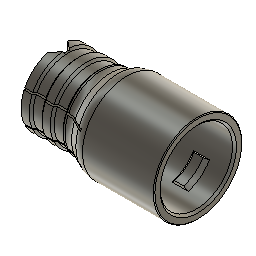
Bosch GEX 40-150 Festool Adapter v2 (Autodesk Fusion 360 design; units mm, degrees)
Autodesk Fusion 360 part; units mm, degrees
sketch "Sketch1" plane through (0, 0, 0) normal (0, 1, 0) x (1, 0, 0)
  line L0 (0, -14.25) -> (25, -14.25)
  line L1 (25, -14.25) -> (33, -18)
  line L2 (33, -18) -> (70, -18)
  line L3 (0, -14.25) -> (0, -18.25)
  line L4 (0, -18.25) -> (24.109, -18.25)
  line L5 (24.109, -18.25) -> (32.109, -22)
  line L6 (32.109, -22) -> (70, -22)
  line L7 (70, -22) -> (70, -18)
  line L8 (52, -18) -> (53.75, -16.25)
  line L9 (53.75, -16.25) -> (58.25, -16.25)
  line L10 (58.25, -16.25) -> (60, -18)
  line L11 (3.8, -5.35) -> (3.8, 5.35)
  arc A0 (3.8, 5.35) -> (0, 5.35) centre (1.9, 5.35) ccw
  line L12 (0, 5.35) -> (0, -5.35)
  arc A1 (0, -5.35) -> (3.8, -5.35) centre (1.9, -5.35) ccw
  line L13 (1.9, -7.25) -> (1.9, 7.25) construction
  line L14 (1.9, -7.25) -> (31.9, -7.25)
  line L15 (31.9, -7.25) -> (31.9, 7.25)
  line L16 (31.9, 7.25) -> (1.9, 7.25)
  line L17 (4.6, -5.35) -> (4.6, 5.35) construction
  arc A2 (4.6, 5.35) -> (-0.8, 5.35) centre (1.9, 5.35) ccw construction
  line L18 (-0.8, 5.35) -> (-0.8, -5.35) construction
  arc A3 (-0.8, -5.35) -> (4.6, -5.35) centre (1.9, -5.35) ccw construction
  line L19 (1.9, -8.05) -> (32.7, -8.05)
  line L20 (32.7, -8.05) -> (32.7, 8.05)
  line L21 (32.7, 8.05) -> (1.9, 8.05)
  line L22 (31.9, -7.25) -> (31.9, -8.05)
  line L23 (31.9, 7.25) -> (31.9, 8.05)
  line L24 (0, -14.25) -> (3.8, -10.45)
  line L25 (3.8, -10.45) -> (3.8, -14.25)
  line L26 (2.8, -11.45) -> (3.8, -11.45)
  line L27 (1.9, -8.05) -> (0, -8.05)
  line L28 (0, 8.05) -> (1.9, 8.05)
  line L29 (0, -8.05) -> (0, -5.35)
  line L30 (0, 8.05) -> (0, 5.35)
  line L31 (1.9, -7.25) -> (0, -7.25)
  line L32 (1.9, 7.25) -> (0, 7.25)
  line L33 (5, -18.25) -> (5, -17.25)
  line L34 (5, -17.25) -> (9.5, -17.25)
  line L35 (9.5, -17.25) -> (9.5, -18.25)
  line L36 (15.5, -18.25) -> (15.5, -17.25)
  line L37 (15.5, -17.25) -> (20, -17.25)
  line L38 (20, -17.25) -> (20, -18.25)
  point P0 (1.9, 0)
  dimension "d1" = 14.25
  dimension "d2" = 4
  dimension "d3" = 25
  dimension "d4" = 18
  dimension "d5" = 4
  dimension "d6" = 4
  dimension "d7" = 8
  dimension "d8" = 135
  dimension "d9" = 1.75
  dimension "d10" = 10
  dimension "d11" = 19
  dimension "d12" = 45
  dimension "d17" = 14.5
  dimension "d18" = 3.8
  dimension "d20" = 30
  dimension "d21" = 0.8
  dimension "d22" = 0.8
  dimension "d24" = 45
  dimension "d27" = 1
  dimension "d34" = 1
  dimension "d35" = 4.5
  dimension "d36" = 6
  dimension "d37" = 5
  constraint horizontal L0
  constraint parallel L0 L2
  constraint perpendicular L0 L3
  constraint perpendicular L3 L4
  constraint parallel L4 L6
  constraint vertical L7
  constraint vertical origin L0.start
  constraint parallel L1 L5
  constraint coincident L2 L8.start
  constraint parallel L2 L9
  constraint coincident L2 L10.end
  constraint equal L8 L10
  constraint tangent L11 A0
  constraint tangent A0 L12
  constraint parallel L11 L12
  constraint tangent L12 A1
  constraint tangent L11 A1
  constraint midpoint A1 L13.start
  constraint midpoint A0 L13.end
  constraint perpendicular L0 L13
  constraint midpoint L13 P0
  constraint horizontal origin P0
  constraint tangent A1 L14
  constraint perpendicular L13 L14
  constraint perpendicular L14 L15
  constraint horizontal L16
  constraint coincident L19 L22.end
  constraint perpendicular L19 L22
  constraint coincident L21 L23.end
  constraint perpendicular L21 L23
  constraint coincident origin L12
  constraint perpendicular L0 L25
  constraint coincident L0 L25.end
  constraint coincident L11 L24.end
  constraint coincident L24 L26.start
  constraint coincident L25 L26.end
  constraint perpendicular L25 L26
  constraint tangent A3 L27
  constraint parallel L19 L27
  constraint tangent A2 L28
  constraint horizontal L28
  constraint vertical L30
  constraint vertical L29
  constraint coincident L29 L31.end
  constraint coincident L30 L32.end
  constraint horizontal L32
  constraint horizontal L31
  constraint coincident L4 L33.start
  constraint perpendicular L4 L33
  constraint perpendicular L33 L34
  constraint coincident L4 L35.end
  constraint coincident L4 L36.start
  constraint perpendicular L4 L36
  constraint perpendicular L36 L37
  constraint coincident L4 L38.end
  constraint parallel L35 L38
  constraint vertical L38
  constraint equal L34 L37
  constraint equal L35 L36
  measures "d1" distance of origin L0
  measures "d2" distance of L0.start L3.end
  measures "d3" distance of L0.start L0.end
  measures "d4" distance of origin L2
  measures "d5" distance of L2 L6
  measures "d6" distance of L1 L5
  measures "d7" distance of L8.start L10.end
  measures "d8" angle of L9 L10
  measures "d9" vertical distance of L9.end L10.end
  measures "d10" distance of L2.end L10.end
  measures "d11" distance of L1.end L8.start
  measures "d12" horizontal distance of L0.end L6.end
  measures "d17" distance of L13.start L13.end
  measures "d18" distance of L11 L12
  measures "d20" distance of L13.end L15.end
  measures "d24" angle of L24 L25
  measures "d27" vertical distance of L24.end L26.start
  measures "d34" distance of L36.start L36.end
  measures "d35" distance of L36.end L37.end
  measures "d36" distance of L34.end L36.end
  measures "d37" distance of L3.end L33.start
revolve "Revolve1" add sketch "Sketch1" angle 360 about axis through (1.75, 0, 0) along (1, 0, 0) contours L0 L1 L2 L3 L4 L5 L6 L7 L33 L34 L35 L36 L37 L38 makes body 1
chamfer "Chamfer2" distance 1 angle 45 4 edges at (5, -6.5995, -17.015) (9.5, -6.5995, -17.015) (15.5, -6.5995, -17.015) (20, -6.5995, -17.015) on bodies 1
revolve "Revolve2" add sketch "Sketch1" angle 44 about axis through (1.75, 0, 0) along (-1, 0, 0) contours L2 L8 L9 L10 bodies 1
sketch "Sketch2" plane through (0, 0, 0) normal (0, 0, 1) x (1, 0, 0)
  line L0 (0, 5.0346) -> (6, 0)
  line L1 (6, 0) -> (0, -5.0346)
  line L2 (0, -5.0346) -> (0, 5.0346)
  dimension "d39" = 80
  dimension "d40" = 6
  constraint vertical L2
  constraint midpoint origin L2
  constraint equal L0 L1
  measures "d39" angle of L0 L1
  measures "d40" distance of origin L0.end
extrude "Extrude3" cut sketch "Sketch2" along normal through all and the other way through all bodies 1
chamfer "Chamfer3" distance 2 angle 45 2 edges at (6, 0, 15.75) (6, 0, -15.75) on bodies 1
fillet "Fillet1" radius 10 4 edges at (24.109, -6.5995, -17.015) (32.109, -7.9555, -20.5112) (25, -5.153, -13.2857) (33, -6.5091, -16.7819) on bodies 1
pattern_circular "C-Pattern1" count 3 over 360 about axis through (1.75, 0, 0) along (1, 0, 0) of "Revolve2"
extrude "Extrude1" cut sketch "Sketch1" along normal through all and the other way through all contours L14 L19 L22 L27 L29 L31 | L16 L21 L23 L28 L30 L32 bodies 1
revolve "Revolve4" add sketch "Sketch1" angle 360 about axis through (1.75, 0, 0) along (1, 0, 0) separate body contours L0 L24 L25 L26 makes body 2
extrude "Extrude2" cut sketch "Sketch1" along normal through all and the other way through all contours L11 A0 L12 A1 keep common part bodies 2 makes body 3 at (0.9333, 13.2866, -0.8945)
chamfer "Chamfer1" distance 1 angle 45 1 edges at (70, -6.5091, -16.7819) on bodies 1
chamfer "Chamfer1" distance 0.4 angle 45 1 edges at (70, -7.9555, -20.5112) on bodies 1
combine "Combine1" operation add target body 1 tool bodies 3 2
equation "d1 = ( 28.5 / 2 ) * 1 mm"
equation "d4 = ( 36 / 2 ) * 1 mm"
equation "d5 = d2"
equation "d6 = d2"
